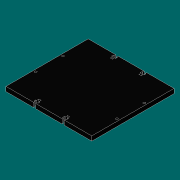
# Autodesk Inventor part: topBottomPanel
Saved by Autodesk Inventor 2016 (Build 200138000, 138)
## iProperties
Created: 2015-10-05
Part Number: topBottomPanel
Material: ABS Plastic
Document SubType Name: Modeling
Designer: sawai
Density: 1.06 g/cm^3
Appearance: Smooth - Black
Author: sawai
Autodesk Inventor part; units mm, degrees
ref_plane "YZ Plane" through (0, 0, 0) normal (1, 0, 0) x (0, 1, 0)
ref_plane "XZ Plane" through (0, 0, 0) normal (0, 1, 0) x (-1, 0, 0)
ref_plane "XY Plane" through (0, 0, 0) normal (0, 0, 1) x (1, 0, 0)
sketch "Sketch1" plane through (0, 0, 0) normal (0, 0, 1) x (1, 0, 0)
  line L0 (-60, -57.5) -> (60, -57.5)
  line L1 (60, -57.5) -> (60, 57.5)
  line L2 (60, 57.5) -> (-60, 57.5)
  line L3 (-60, 57.5) -> (-60, -57.5)
  line L4 (-60, -57.5) -> (60, 57.5) construction
  line L5 (60, -57.5) -> (-60, 57.5) construction
  point P0 (0, 0)
  dimension "d0" = 120
  dimension "d1" = 115
  constraints: 12 end point, 2 midpoint, 2 parallel, 1 horizontal, 1 perpendicular
  measures "d0" distance of L2.end L1.end
  measures "d1" distance of L1.end L0.end
extrude "Extrusion1" add sketch "Sketch1" along normal blind 6.35
sketch "Sketch3" plane through (0, 0, 6.35) normal (0, 0, 1) x (1, 0, 0)
  line L0 (-60, -57.5) -> (60, -57.5) projected
  line L1 (60, -57.5) -> (60, 57.5) projected
  line L2 (60, 57.5) -> (-60, 57.5) projected
  line L3 (-60, 57.5) -> (-60, -57.5) projected
  line L4 (-56.825, 19.1667) -> (-56.825, -19.1667)
  line L5 (-56.825, -19.1667) -> (56.825, -19.1667)
  line L6 (56.825, -19.1667) -> (56.825, 19.1667)
  line L7 (56.825, 19.1667) -> (-56.825, 19.1667)
  line L8 (-56.825, 19.1667) -> (-56.825, 57.5)
  line L9 (60, 57.5) -> (-60, 57.5) projected
  line L10 (56.825, 19.1667) -> (56.825, 57.5)
  line L11 (56.825, -19.1667) -> (56.825, -57.5)
  line L12 (-60, -57.5) -> (60, -57.5) projected
  line L13 (-56.825, -19.1667) -> (-56.825, -57.5)
  point P0 (0, 0)
  dimension "d4" = 3.175
  dimension "d5" = 3.175
  constraints: 16 end point, 4 point on line, 3 vertical, 2 collinear, 2 horizontal, 2 parallel, 1 perpendicular
  measures "d4" distance between parallel lines of L3 L4
  measures "d5" distance between parallel lines of L1 L6
hole "Hole1" at (-56.825, 19.1667, 6.35) at (-56.825, -19.1667, 6.35) at (56.825, -19.1667, 6.35) at (56.825, 19.1667, 6.35) direction (0, 0, -1) diameter 3 end through all
sketch "Sketch4" plane through (0, 0, 6.35) normal (0, 0, 1) x (1, 0, 0)
  circle A0 centre (56.825, -19.1667) radius 1.5 projected
  circle A1 centre (-56.825, 19.1667) radius 1.5 projected
  circle A2 centre (-56.825, -19.1667) radius 1.5 projected
  circle A3 centre (56.825, 19.1667) radius 1.5 projected
  line L0 (-60, -57.5) -> (60, -57.5) projected
  line L1 (60, -57.5) -> (60, 57.5) projected
  line L2 (60, 57.5) -> (-60, 57.5) projected
  line L3 (-60, 57.5) -> (-60, -57.5) projected
  line L4 (-21.5, -57.5) -> (-21.5, -55.5)
  line L5 (-21.5, -55.5) -> (-22.75, -55.5)
  line L6 (-22.75, -55.5) -> (-22.75, -53)
  line L7 (-22.75, -53) -> (-21.5, -53)
  line L8 (-21.5, -53) -> (-21.5, -49.85)
  line L9 (-21.5, -49.85) -> (-18.5, -49.85)
  line L10 (-18.5, -49.85) -> (-18.5, -53)
  line L11 (-18.5, -53) -> (-17.25, -53)
  line L12 (-17.25, -53) -> (-17.25, -55.5)
  line L13 (-17.25, -55.5) -> (-18.5, -55.5)
  line L14 (-18.5, -55.5) -> (-18.5, -57.5)
  point P0 (0, 0)
  point P1 (-20, -49.85)
  dimension "d13" = 3
  dimension "d14" = 2.5
  dimension "d15" = 5.5
  dimension "d16" = 2
  dimension "d17" = 7.65
  dimension "d18" = 40
  constraints: 22 end point, 10 point on line, 6 perpendicular, 1 collinear, 1 midpoint, 1 vertical
  measures "d13" distance between parallel lines of L14 L4
  measures "d14" distance between parallel lines of L5 L7
  measures "d15" distance between parallel lines of L12 L6
  measures "d16" distance between parallel lines of L0 L5
  measures "d17" distance between parallel lines of L0 L9
  measures "d18" distance from line of L3 point (-20, -49.85)
extrude "Extrusion2" cut sketch "Sketch4" against normal through all contours L4 L5 L6 L7 L8 L9 L10 L11 L12 L13 L14 L0
pattern_linear "Rectangular Pattern1" count 2 spacing 40 along (1, 0, 0) of "Extrusion2"
mirror "Mirror1" about plane through (0, 0, 0) normal (0, 1, 0) of "Extrusion2", "Rectangular Pattern1"
equation "\"d0\" = width"
equation "\"d1\" = depth"
equation "\"d2\" = materialThickness"
equation "\"d4\" = 0.5 * materialThickness"
equation "\"d5\" = 0.5 * materialThickness"
equation "\"d14\" = nutTrapDepth"
equation "\"d15\" = nutTrapwidth"
equation "\"d16\" = nutTrapClearence"
equation "\"d18\" = 0.333333 * width"
equation "\"d23\" = 0.333333 * width"
equation "\"width\" = 120"
equation "\"depth\" = 115"
equation "\"materialThickness\" = 6.35"
equation "\"laserKerf\" = 0.1"
equation "\"spoolDiameter\" = 95"
equation "\"cardPinDiameter\" = 3"
equation "\"cardFillet\" = 2.88"
equation "\"cardSelected\" = 1"
equation "\"cardThickness\" = 0.76"
equation "\"cardHeight\" = 53.98"
equation "\"cardWidth\" = 85.6"
equation "\"centeralShaftDiameter\" = 8"
equation "\"cardClearence\" = 0.5"
equation "\"bearingOd\" = 22"
equation "\"bearingWidth\" = 8"
equation "\"axleHeight\" = 95"
equation "\"nutTrapDepth\" = 2.5"
equation "\"nutTrapwidth\" = 5.5"
equation "\"nutTrapClearence\" = 2"
equation "\"magnetDiameter\" = 6"
equation "\"magnetProtusion\" = 0.25"
body "Solid1"
